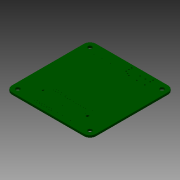
# Autodesk Inventor part: PQ60 Radio FV1.brd_Outline
Saved by Autodesk Inventor 2015 SP1 (Build 190203100, 203)
## iProperties
Created: 2015-10-19
Part Number: PQ60 Radio FV1.brd_Outline
Material: Generic
Document SubType Name: Modeling
Designer: Kartikye
Density: 1 g/cm^3
Appearance: Board Outline
Author: Kartikye
Autodesk Inventor part; units mm, degrees
ref_plane "YZ Plane" through (0, 0, 0) normal (1, 0, 0) x (0, 1, 0)
ref_plane "XZ Plane" through (0, 0, 0) normal (0, 1, 0) x (-1, 0, 0)
ref_plane "XY Plane" through (0, 0, 0) normal (0, 0, 1) x (1, 0, 0)
sketch "Sketch1" plane through (0, 0, 0) normal (0, 0, 1) x (1, 0, 0)
  line L0 (42, 3) -> (42, 39)
  line L1 (42, 39) -> (41.8978, 39.7765)
  line L2 (41.8978, 39.7765) -> (41.5981, 40.5)
  line L3 (41.5981, 40.5) -> (41.1213, 41.1213)
  line L4 (41.1213, 41.1213) -> (40.5, 41.5981)
  line L5 (40.5, 41.5981) -> (39.7765, 41.8978)
  line L6 (39.7765, 41.8978) -> (39, 42)
  line L7 (39, 42) -> (3, 42)
  line L8 (3, 42) -> (2.2235, 41.8978)
  line L9 (2.2235, 41.8978) -> (1.5, 41.5981)
  line L10 (1.5, 41.5981) -> (0.8787, 41.1213)
  line L11 (0.8787, 41.1213) -> (0.4019, 40.5)
  line L12 (0.4019, 40.5) -> (0.1022, 39.7765)
  line L13 (0.1022, 39.7765) -> (0, 39)
  line L14 (0, 39) -> (0, 3)
  line L15 (0, 3) -> (0.1022, 2.2235)
  line L16 (0.1022, 2.2235) -> (0.4019, 1.5)
  line L17 (0.4019, 1.5) -> (0.8787, 0.8787)
  line L18 (0.8787, 0.8787) -> (1.5, 0.4019)
  line L19 (1.5, 0.4019) -> (2.2235, 0.1022)
  line L20 (2.2235, 0.1022) -> (3, 0)
  line L21 (3, 0) -> (39, 0)
  line L22 (39, 0) -> (39.7765, 0.1022)
  line L23 (39.7765, 0.1022) -> (40.5, 0.4019)
  line L24 (40.5, 0.4019) -> (41.1213, 0.8787)
  line L25 (41.1213, 0.8787) -> (41.5981, 1.5)
  line L26 (41.5981, 1.5) -> (41.8978, 2.2235)
  line L27 (41.8978, 2.2235) -> (42, 3)
  circle A0 centre (32.1, 8.8) radius 0.55
  circle A1 centre (9.9, 8.8) radius 0.35
  circle A2 centre (32.1, 8.5) radius 0.55
  circle A3 centre (9.9, 8.5) radius 0.35
  circle A4 centre (14.1, 12.3) radius 0.15
  circle A5 centre (29.7, 2.45) radius 0.15
  circle A6 centre (30.6, 9.2) radius 0.15
  circle A7 centre (27.3, 11.3) radius 0.15
  circle A8 centre (24.9, 11.3) radius 0.15
  circle A9 centre (23.1, 2.6) radius 0.15
  circle A10 centre (22.5, 11.3) radius 0.15
  circle A11 centre (19.5, 11.3) radius 0.15
  circle A12 centre (17.7, 12.3) radius 0.15
  circle A13 centre (3, 3) radius 1
  circle A14 centre (3, 39) radius 1
  circle A15 centre (39, 39) radius 1
  circle A16 centre (39, 3) radius 1
  circle A17 centre (20.7, 1.9) radius 0.15
  circle A18 centre (25.5, 2.6) radius 0.15
  circle A19 centre (21.3, 7) radius 0.15
  circle A20 centre (13.5, 11.3) radius 0.15
  circle A21 centre (15.9, 11.3) radius 0.15
  circle A22 centre (18.3, 11.3) radius 0.15
  circle A23 centre (20.7, 11.3) radius 0.15
  circle A24 centre (23.7, 11.3) radius 0.15
  circle A25 centre (26.1, 11.3) radius 0.15
  circle A26 centre (28.5, 11.3) radius 0.15
  circle A27 centre (15.3, 12.3) radius 0.15
  circle A28 centre (14.7, 11.3) radius 0.15
  circle A29 centre (14.1, 2.7) radius 0.15
  circle A30 centre (14.7, 1.9) radius 0.15
  circle A31 centre (15.3, 2.7) radius 0.15
  circle A32 centre (15.9, 1.9) radius 0.15
  circle A33 centre (16.5, 2.7) radius 0.15
  circle A34 centre (17.1, 1.9) radius 0.15
  circle A35 centre (17.7, 2.7) radius 0.15
  circle A36 centre (18.3, 1.9) radius 0.15
  circle A37 centre (31, 12.2) radius 0.15
  circle A38 centre (18.9, 2.7) radius 0.15
  circle A39 centre (19.5, 1.9) radius 0.15
  circle A40 centre (20.1, 2.7) radius 0.15
  circle A41 centre (12.9, 2.7) radius 0.15
  circle A42 centre (15, 37.1) radius 0.15
  circle A43 centre (12.3, 1.9) radius 0.15
  circle A44 centre (11, 37) radius 0.15
  circle A45 centre (22.4, 40.5) radius 0.3
  circle A46 centre (22.4, 39.1) radius 0.3
  circle A47 centre (22.4, 37.7) radius 0.3
  circle A48 centre (23.7, 37.1) radius 0.3
  circle A49 centre (25, 36.4) radius 0.3
  circle A50 centre (29, 36.4) radius 0.3
  circle A51 centre (28, 39.1) radius 0.3
  circle A52 centre (30.6, 39.1) radius 0.3
  circle A53 centre (33, 40.5) radius 0.3
  circle A54 centre (33, 39.1) radius 0.3
  circle A55 centre (33, 36.4) radius 0.3
  circle A56 centre (13.5, 1.9) radius 0.15
  circle A57 centre (7, 37) radius 0.15
  circle A58 centre (12.9, 12.3) radius 0.15
  circle A59 centre (12.3, 11.3) radius 0.15
  constraints: 60 centre point, 56 end point
extrude "PQ60 Radio FV1.brd_Outline" add sketch "Sketch1" along normal blind 1
body "Solid1"
